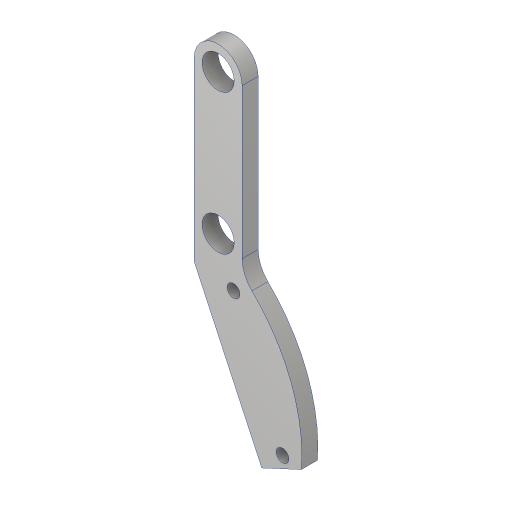
# Autodesk Inventor part: Grip_
Saved by Autodesk Inventor 2023.2 (Build 272271000, 271)
## iProperties
Created: 2021-07-28
Part Number: Grip_
Material: 알루미늄 6061
Document SubType Name: Modeling
Designer: user
Density: 2.7 g/cm^3
Appearance: 알루미늄 - 평지
Mass: 10.8393 g
Surface Area: 30.9529 cm^2
Volume: 4.01455 cm^3
Author: user
Autodesk Inventor part; units mm, degrees
ref_plane "YZ Plane" through (0, 0, 0) normal (1, 0, 0) x (0, 1, 0)
ref_plane "XZ Plane" through (0, 0, 0) normal (0, 1, 0) x (-1, 0, 0)
ref_plane "XY Plane" through (0, 0, 0) normal (0, 0, 1) x (1, 0, 0)
sketch "스케치1" plane through (0, 0, 0) normal (0, 0, 1) x (1, 0, 0)
  line L0 (0, 0) -> (8.4524, -18.1262)
  line L1 (0, 0) -> (20, 0) construction
  line L2 (8.4524, -18.1262) -> (14.7965, -15.1678)
  line L3 (8.4524, -18.1262) -> (16.9047, -36.2523)
  line L4 (8.4524, -18.1262) -> (28.4524, -18.1262) construction
  arc A0 (16.9047, -36.2523) -> (0, 0) centre (-14.2701, -28.7218) ccw
  line L5 (0, 0) -> (0, 50)
  line L6 (0, 0) -> (50, 0) construction
  line L7 (0, 50) -> (12, 50)
  line L8 (12, 50) -> (12, 3)
  circle A1 centre (6, 44) radius 4.025
  circle A2 centre (6, 9) radius 4.025
  line L9 (16.9047, -36.2523) -> (26.8143, -31.6314)
  line L10 (16.9047, -36.2523) -> (27.8387, -36.2523) construction
  line L11 (12, -47.3039) -> (11.9482, -47.1928)
  arc A3 (26.2229, -36.2523) -> (12, 3) centre (-14.2701, -28.7218) ccw
  dimension "d16" = 20
  dimension "d17" = 65
  dimension "d18" = 7
  dimension "d19" = 90
  dimension "d20" = 20
  dimension "d21" = 65
  dimension "d22" = 50
  dimension "d23" = 90
  dimension "d24" = 12
  dimension "d25" = 90
  dimension "d26" = 47
  dimension "d27" = 8.05
  dimension "d28" = 8.05
  dimension "d29" = 6
  dimension "d30" = 6
  dimension "d31" = 6
  dimension "d32" = 35
  dimension "d33" = 25
  constraints: 24 end point, 7 point on circle, 4 centre point, 4 equal length, 4 horizontal, 3 perpendicular, 2 point on line, 1 vertical
  measures "d16" distance of L0.start L0.end
  measures "d17" angle of L0 L1
  measures "d18" distance of L0.end L2.end
  measures "d19" angle of L2 L0
  measures "d20" distance of L0.end L3.end
  measures "d21" angle of L3 L4
  measures "d22" distance of L0.start L5.end
  measures "d23" angle of L6 L5
  measures "d24" distance of L5.end L7.end
  measures "d25" angle of L5 L7
  measures "d26" distance of L7.end L8.end
  measures "d27" diameter of A1
  measures "d28" diameter of A2
  measures "d29" distance from line of L7 A1.centre
  measures "d30" distance from line of L8 A1.centre
  measures "d31" distance from line of L8 A2.centre
  measures "d32" distance of A1.centre A2.centre
  measures "d33" angle of L10 L9
extrude "돌출1" add sketch "스케치1" along normal blind 4 contours L5 L7 L8 A3 L9 A0
fillet "모깎기1" radius 6 2 edges at (12, 50, 2) (0, 50, 2)
sketch "스케치2" plane through (0, 0, 4) normal (0, 0, 1) x (1, 0, 0)
  line L0 (16.9047, -36.2523) -> (26.8143, -31.6314) projected
  arc A0 (17.3077, -34.3271) -> (18.715, -35.4082) centre (18.2923, -34.5019) ccw projected
  arc A1 (26.2765, -31.8822) -> (26.8523, -31.032) centre (25.8539, -30.9759) ccw projected
  line L1 (20, -34.809) -> (17.8869, -30.2774)
  line L2 (20, -34.809) -> (25, -34.809) construction
  line L3 (17.8869, -30.2774) -> (26.834, -26.1053)
  arc A2 (26.8143, -31.6314) -> (12, 3) centre (-14.2701, -28.7218) ccw projected
  line L4 (26.834, -26.1053) -> (17.7607, -30.3363)
  arc A3 (16.9047, -36.2523) -> (0, 0) centre (-14.2701, -28.7218) ccw projected
  arc A4 (26.2765, -31.8822) -> (26.8523, -31.032) centre (25.8539, -30.9759) ccw projected
  line L5 (26.834, -26.1053) -> (16.9047, -36.2523)
  line L6 (17.7607, -30.3363) -> (26.8143, -31.6314)
  circle A5 centre (22.0881, -30.9553) radius 1.6
  point P0 (12.3536, 2.7038)
  point P1 (0.5383, -0.2738)
  dimension "d38" = 5
  dimension "d39" = 115
  dimension "d40" = 90
  dimension "d41" = 3.2
  constraints: 12 end point, 4 point on line, 2 point on circle, 1 centre point, 1 equal length, 1 horizontal
  measures "d38" distance of L1.start L1.end
  measures "d39" angle of L2 L1
  measures "d40" angle of L1 L3
  measures "d41" diameter of A5
extrude "돌출2" cut sketch "스케치2" against normal blind 4 contours A5 L6 L5 | L5 L6 A5 | A5 L5 L6 | L5 A5 L6
sketch "스케치4" plane through (0, 0, 4) normal (0, 0, 1) x (1, 0, 0)
  line L0 (12, 3) -> (12, 44) projected
  line L1 (12, 3) -> (2.5423, -1.4102)
  arc A0 (16.9047, -36.2523) -> (0, 0) centre (-14.2701, -28.7218) ccw projected
  line L2 (12, 3) -> (22.4355, 3) construction
  line L3 (7.2711, 0.7949) -> (9.8068, -4.643)
  line L4 (7.2711, 0.7949) -> (13.2711, 0.7949) construction
  line L5 (9.8068, -4.643) -> (7.8894, -5.5371)
  line L6 (9.8068, -4.643) -> (16.6121, -1.4696)
  arc A1 (26.8143, -31.6314) -> (12, 3) centre (-14.2701, -28.7218) ccw projected
  line L7 (9.8068, -4.643) -> (17.3156, -4.643) construction
  line L8 (2.5423, -1.4102) -> (16.6121, -1.4696)
  line L9 (7.8894, -5.5371) -> (12, 3)
  circle A2 centre (9.8616, -1.4411) radius 1.6
  dimension "d54" = 155
  dimension "d55" = 6
  dimension "d57" = 25
  dimension "d58" = 3.2
  constraints: 18 end point, 3 equal length, 3 horizontal, 3 point on circle, 2 perpendicular, 2 point on line, 1 centre point, 1 midpoint
  measures "d54" angle of L1 L2
  measures "d55" distance of L3.start L3.end
  measures "d57" angle of L7 L6
  measures "d58" diameter of A2
extrude "돌출4" cut sketch "스케치4" against normal up to surface (4 mm away) contours A2 L8 L9 | L9 L8 L3 A2 | L3 L8 A2 | A2 L9 L8 | L9 A2 L3 L8 | L8 L3 A2
sketch "스케치6" plane through (0, 0, 0) normal (0, 0, -1) x (-1, 0, 0)
  arc A0 (0, 0) -> (-16.9047, -36.2523) centre (14.2701, -28.7218) ccw projected
  line L0 (0, 0) -> (-16.9047, -36.2523)
  line L1 (-16.9047, -36.2523) -> (-26.8143, -31.6314) projected
  line L2 (-16.9047, -36.2523) -> (-26.8143, -31.6314)
  line L3 (-26.8143, -31.6314) -> (-9.9095, 4.6209)
  line L4 (-9.9095, 4.6209) -> (0, 0)
  constraints: 8 end point, 1 collinear, 1 perpendicular
extrude "돌출6" add sketch "스케치6" against normal up to surface (4 mm away) contours L0 A0
fillet "모깎기3" radius 8 1 edges at (12, 3, 2)
